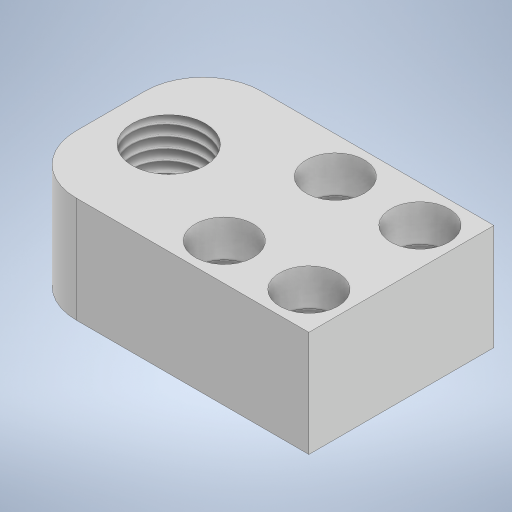
# Autodesk Inventor part: Spindlesocket
Saved by Autodesk Inventor 2024 (Build 280153000, 153)
## iProperties
Created: 2023-05-10
Part Number: Spindlesocket
Material: Generic
Document SubType Name: Modeling
Designer: dell
Density: 1 g/cm^3
Appearance: Default
Author: dell
Autodesk Inventor part; units mm, degrees
ref_plane "YZ Plane" through (0, 0, 0) normal (1, 0, 0) x (0, 1, 0)
ref_plane "XZ Plane" through (0, 0, 0) normal (0, 1, 0) x (-1, 0, 0)
ref_plane "XY Plane" through (0, 0, 0) normal (0, 0, 1) x (1, 0, 0)
sketch "Sketch1" plane through (0, 0, 0) normal (0, 1, 0) x (-1, 0, 0)
  line L0 (27.5, 17.5) -> (-27.5, 17.5)
  line L1 (-27.5, 17.5) -> (-27.5, -17.5)
  line L2 (-27.5, -17.5) -> (27.5, -17.5)
  line L3 (27.5, -17.5) -> (27.5, 17.5)
  line L4 (27.5, 17.5) -> (-27.5, -17.5) construction
  line L5 (-27.5, 17.5) -> (27.5, -17.5) construction
  point P0 (0, 0)
  dimension "d0" = 55
  dimension "d1" = 35
  constraints: 12 end point, 2 midpoint, 2 parallel, 1 horizontal, 1 perpendicular
  measures "d0" distance of L1.end L2.end
  measures "d1" distance of L2.end L0.start
extrude "Extrusion1" add sketch "Sketch1" along normal blind 20
sketch "Sketch2" plane through (0, 20, 0) normal (0, 1, 0) x (1, 0, 0)
  circle A0 centre (20.5, 10.5) radius 5.5
  circle A1 centre (20.5, -10.5) radius 5.5
  circle A2 centre (4.5, -10.5) radius 5.5
  circle A3 centre (4.5, 10.5) radius 5.5
  line L0 (27.5, -17.5) -> (27.5, 17.5) projected
  point P0 (0, 0)
  dimension "d4" = 11
  dimension "d5" = 11
  dimension "d6" = 11
  dimension "d7" = 11
  dimension "d8" = 21
  dimension "d9" = 21
  dimension "d10" = 10.5
  dimension "d11" = 10.5
  dimension "d12" = 23
  dimension "d13" = 23
  dimension "d14" = 7
  dimension "d15" = 7
  constraints: 4 centre point
  measures "d4" diameter of A3
  measures "d5" diameter of A0
  measures "d6" diameter of A2
  measures "d7" diameter of A1
  measures "d8" distance of A1.centre A0.centre
  measures "d9" distance of A2.centre A3.centre
  measures "d10" vertical distance of point (0, 0) A3.centre
  measures "d11" vertical distance of point (0, 0) A0.centre
  measures "d12" distance from line of L0 A2.centre
  measures "d13" distance from line of L0 A3.centre
  measures "d14" distance from line of L0 A0.centre
  measures "d15" distance from line of L0 A1.centre
extrude "Extrusion2" cut sketch "Sketch2" against normal blind 7
sketch "Sketch3" plane through (4.5, 13, 10.5) normal (0, 1, 0) x (1, 0, 0)
  circle A0 centre (0, 0) radius 3.2
  circle A1 centre (0, 21) radius 5.5 projected
  circle A2 centre (16, 21) radius 5.5 projected
  circle A3 centre (16, 0) radius 5.5 projected
  circle A4 centre (0, 21) radius 3.2
  circle A5 centre (16, 21) radius 3.2
  circle A6 centre (16, 0) radius 3.2
  point P0 (-4.5, 10.5)
  dimension "d18" = 6.4
  dimension "d19" = 6.4
  dimension "d20" = 6.4
  dimension "d21" = 6.4
  constraints: 4 centre point, 3 coincident
  measures "d18" diameter of A4
  measures "d19" diameter of A0
  measures "d20" diameter of A5
  measures "d21" diameter of A6
extrude "Extrusion3" cut sketch "Sketch3" against normal blind 20 contours A0 | A4 | A5 | A6
sketch "Sketch4" plane through (0, 20, 0) normal (0, 1, 0) x (1, 0, 0)
  line L0 (27.5, -17.5) -> (27.5, 17.5) projected
  point P0 (0, 0)
  point P1 (-16.5, 0)
  dimension "d27" = 44
  measures "d27" distance from line of L0 point (-16.5, 0)
fillet "Fillet1" radius 11 2 edges at (-27.5, 10, 17.5) (-27.5, 10, -17.5)
hole "Hole1" at (-16.5, 20, 0) direction (0, -1, 0) diameter 13.835 depth 41.3 thread size "M16x2" class "6H" standard "ISO Metric profile"
body "Solid1"
